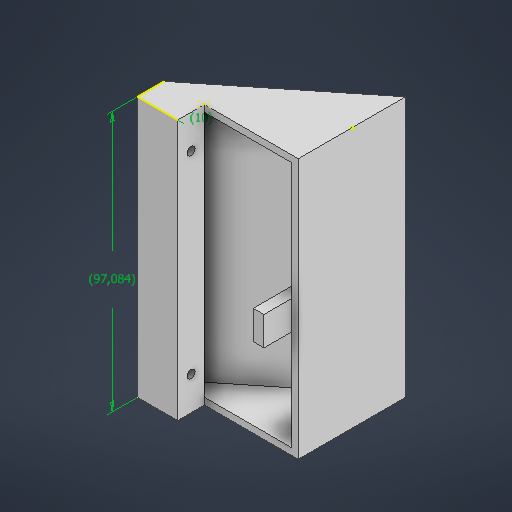
# Autodesk Inventor part: Rampa 1
Saved by Autodesk Inventor 2026.1 (Build 301233020, 233B)
## iProperties
Created: 2025-11-07
Part Number: Rampa 1
Material: Genérico
Document SubType Name: Modeling
Designer: david
Density: 1 g/cm^3
Appearance: Padrão
Author: david
Autodesk Inventor part; units mm, degrees
ref_plane "YZ Plane" through (0, 0, 0) normal (1, 0, 0) x (0, 1, 0)
ref_plane "XZ Plane" through (0, 0, 0) normal (0, 1, 0) x (-1, 0, 0)
ref_plane "XY Plane" through (0, 0, 0) normal (0, 0, 1) x (1, 0, 0)
sketch "Esboço1" plane through (0, 0, 0) normal (0, 1, 0) x (-1, 0, 0)
  line L0 (0, 20) -> (0, -20)
  line L1 (0, 20) -> (50, 20)
  line L2 (50, 20) -> (0, -20)
  line L3 (50, 20) -> (50, 30)
  line L4 (50, 30) -> (35, 30)
  line L5 (35, 30) -> (35, 20)
  point P0 (0, 0)
  dimension "d0" = 40
  dimension "d1" = 50
  dimension "d2" = 10
  dimension "d3" = 15
  constraints: 12 end point, 2 horizontal, 2 perpendicular, 1 midpoint, 1 point on line, 1 vertical
  measures "d0" distance of L0.start L0.end
  measures "d1" distance of L0.start L1.end
  measures "d2" distance of L1.end L3.end
  measures "d3" distance of L3.end L4.end
extrude "Extrusão1" add sketch "Esboço1" along normal blind 97.084
shell "Casca1" thickness 2.5 removed faces 1 at (-23.3333, 32.3613, 20)
sketch "Esboço2" plane through (-50, 0, 20) normal (-1, 0, 0) x (0, 0, 1)
  line L0 (10, 97.084) -> (0, 97.084) projected
  line L1 (0, 97.084) -> (5, 97.084)
  line L2 (5, 97.084) -> (5, 84.584)
  circle A0 centre (5, 84.584) radius 1.5
  line L3 (10, 0) -> (0, 0) projected
  line L4 (0, 0) -> (5, 0)
  line L5 (5, 0) -> (5, 12.5)
  circle A1 centre (5, 12.5) radius 1.5
  point P0 (-20, 0)
  dimension "d7" = 5
  dimension "d8" = 12.5
  dimension "d9" = 3
  dimension "d10" = 5
  dimension "d11" = 12.5
  dimension "d12" = 3
  constraints: 8 end point, 2 centre point, 2 coincident, 2 midpoint, 2 perpendicular
  measures "d7" distance of L0.end L1.end
  measures "d8" distance of L1.end L2.end
  measures "d9" diameter of A0
  measures "d10" distance of L3.end L4.end
  measures "d11" distance of L4.end L5.end
  measures "d12" diameter of A1
extrude "Extrusão2" cut sketch "Esboço2" against normal blind 102.84
thread "Rosca1" size "M3x0.5" class "6H" standard "ANSI Metric M Profile" length 20
thread "Rosca2" size "M3x0.5" class "6H" standard "ANSI Metric M Profile" length 20
thread "Rosca3" size "M3x0.5" class "6H" standard "ANSI Metric M Profile" length 20
thread "Rosca4" size "M3x0.5" class "6H" standard "ANSI Metric M Profile" length 20
sketch "Esboço3" plane through (0, 97.084, 0) normal (0, 1, 0) x (1, 0, 0)
  line L0 (-50, -30) -> (-35, -30) projected
  point P0 (0, 0)
  point P1 (-35, -20)
  dimension "d23" = 10
  measures "d23" distance from line of point (-35, -20) L0
sketch "Esboço4" plane through (-50, 0, 20) normal (-1, 0, 0) x (0, 0, 1)
  line L0 (0, 97.084) -> (10, 97.084) projected
  line L1 (0, 0) -> (10, 0) projected
  point P0 (-20, 0)
  dimension "d24" = 97.084
  measures "d24" distance between parallel lines of L0 L1
sketch "Esboço5" plane through (0, 97.084, 0) normal (0, 1, 0) x (1, 0, 0)
  point P0 (0, 0)
sketch "Esboço6" plane through (-2.5, 2.5, 20) normal (-1, 0, 0) x (0, 0, 1)
  line L0 (-10.2933, 37.3647) -> (10.2933, 37.3647)
  line L1 (10.2933, 37.3647) -> (10.2933, 48.1592)
  line L2 (10.2933, 48.1592) -> (-10.2933, 48.1592)
  line L3 (-10.2933, 48.1592) -> (-10.2933, 37.3647)
  line L4 (0, 92.084) -> (0, 0) projected
  line L5 (-10.2933, 37.3647) -> (10.2933, 48.1592) construction
  line L6 (10.2933, 37.3647) -> (-10.2933, 48.1592) construction
  point P0 (-20, -2.5)
  point P1 (0, 42.762)
  constraints: 12 end point, 2 midpoint, 2 parallel, 1 horizontal, 1 perpendicular, 1 point on line
extrude "Extrusão3" add sketch "Esboço6" along normal blind 4
sketch "Esboço7" plane through (-6.5, 2.5, 20) normal (-1, 0, 0) x (0, 0, 1)
  line L0 (-10.2933, 48.1592) -> (-10.2933, 37.3647) projected
  line L1 (-10.2933, 42.762) -> (-6.2933, 42.762)
  line L2 (10.2933, 37.3647) -> (10.2933, 48.1592) projected
  line L3 (10.2933, 42.762) -> (6.2933, 42.762)
  circle A0 centre (-6.2933, 42.762) radius 1.5
  circle A1 centre (6.2933, 42.762) radius 1.5
  point P0 (-20, -2.5)
  dimension "d27" = 4
  dimension "d28" = 4
  dimension "d29" = 3
  dimension "d30" = 3
  constraints: 4 end point, 2 centre point, 2 coincident, 2 horizontal, 2 midpoint
  measures "d27" distance of L1.start L1.end
  measures "d28" distance of L3.start L3.end
  measures "d29" diameter of A0
  measures "d30" diameter of A1
extrude "Extrusão4" cut sketch "Esboço7" against normal blind 3.5
thread "Rosca5" size "M3x0.5" class "6H" standard "ANSI Metric M Profile" length 20
thread "Rosca6" size "M3x0.5" class "6H" standard "ANSI Metric M Profile" length 20
